Autodesk Fusion 360 part; units mm, degrees
(part 2 of 3)
  spline S12 degree 5 poles (-8.8189, 22.5399) (-8.8218, 22.5475) (-8.8279, 22.5625) (-8.8376, 22.585) (-8.8513, 22.6144) (-8.8698, 22.6507) (-8.8891, 22.6866) (-8.909, 22.7223) (-8.9293, 22.7578) (-8.9498, 22.7932) (-8.9704, 22.8286) (-8.9914, 22.8638) (-9.0127, 22.8988) (-9.0344, 22.9337) (-9.0566, 22.9684) (-9.0792, 23.0028) (-9.1021, 23.0371) (-9.1253, 23.0713) (-9.1488, 23.1053) (-9.1725, 23.1393) (-9.1964, 23.1731) (-9.2206, 23.2068) (-9.245, 23.2403) (-9.2697, 23.2738) (-9.2947, 23.3071) (-9.3199, 23.3403) (-9.3454, 23.3733) (-9.371, 23.4063) (-9.3969, 23.4391) (-9.4231, 23.4718) (-9.4494, 23.5045) (-9.4759, 23.537) (-9.5026, 23.5694) (-9.5296, 23.6016) (-9.5567, 23.6338) (-9.5841, 23.6659) (-9.6117, 23.6978) (-9.6394, 23.7297) (-9.6673, 23.7614) (-9.6955, 23.7931) (-9.7238, 23.8246) (-9.7523, 23.8561) (-9.781, 23.8874) (-9.8098, 23.9186) (-9.8389, 23.9498) (-9.8681, 23.9808) (-9.8974, 24.0117) (-9.927, 24.0425) (-9.9567, 24.0733) (-9.9866, 24.1039) (-10.0167, 24.1344) (-10.0469, 24.1649) (-10.0773, 24.1952) (-10.1079, 24.2254) (-10.1386, 24.2556) (-10.1695, 24.2856) (-10.2005, 24.3156) (-10.2317, 24.3454) (-10.263, 24.3752) (-10.2945, 24.4048) (-10.3262, 24.4344) (-10.358, 24.4639) (-10.3899, 24.4932) (-10.422, 24.5225) (-10.4543, 24.5517) (-10.4867, 24.5808) (-10.5192, 24.6098) (-10.5519, 24.6387) (-10.5847, 24.6675) (-10.6177, 24.6962) (-10.6508, 24.7248) (-10.6774, 24.7476) (-10.6974, 24.7647) (-10.7108, 24.7761) (-10.7175, 24.7818) knots 0 0 0 0 0 0 0.01428571 0.02857143 0.04285714 0.05714286 0.07142857 0.08571429 0.1 0.11428571 0.12857143 0.14285714 0.15714286 0.17142857 0.18571429 0.2 0.21428571 0.22857143 0.24285714 0.25714286 0.27142857 0.28571429 0.3 0.31428571 0.32857143 0.34285714 0.35714286 0.37142857 0.38571429 0.4 0.41428571 0.42857143 0.44285714 0.45714286 0.47142857 0.48571429 0.5 0.51428571 0.52857143 0.54285714 0.55714286 0.57142857 0.58571429 0.6 0.61428571 0.62857143 0.64285714 0.65714286 0.67142857 0.68571429 0.7 0.71428571 0.72857143 0.74285714 0.75714286 0.77142857 0.78571429 0.8 0.81428571 0.82857143 0.84285714 0.85714286 0.87142857 0.88571429 0.9 0.91428571 0.92857143 0.94285714 0.95714286 0.97142857 0.98571429 1 1 1 1 1 1
  arc A26 (-10.7175, 24.7818) -> (-12.2631, 24.0545) centre (0, 0) ccw
  spline S13 degree 5 poles (-11.7459, 21.1625) (-11.7499, 21.1696) (-11.7576, 21.184) (-11.7687, 21.2057) (-11.7827, 21.235) (-11.7989, 21.2724) (-11.8142, 21.3102) (-11.829, 21.3483) (-11.8434, 21.3865) (-11.8577, 21.4248) (-11.8717, 21.4633) (-11.8855, 21.5019) (-11.899, 21.5407) (-11.912, 21.5796) (-11.9245, 21.6188) (-11.9367, 21.6582) (-11.9485, 21.6977) (-11.96, 21.7374) (-11.9713, 21.7771) (-11.9823, 21.817) (-11.9931, 21.857) (-12.0037, 21.8971) (-12.014, 21.9374) (-12.024, 21.9777) (-12.0338, 22.0182) (-12.0433, 22.0588) (-12.0525, 22.0995) (-12.0615, 22.1402) (-12.0703, 22.1811) (-12.0789, 22.2221) (-12.0872, 22.2632) (-12.0954, 22.3043) (-12.1033, 22.3456) (-12.111, 22.3869) (-12.1185, 22.4284) (-12.1257, 22.4699) (-12.1328, 22.5115) (-12.1396, 22.5532) (-12.1463, 22.5949) (-12.1528, 22.6368) (-12.159, 22.6787) (-12.1651, 22.7207) (-12.1709, 22.7628) (-12.1766, 22.8049) (-12.1821, 22.8471) (-12.1874, 22.8894) (-12.1925, 22.9318) (-12.1974, 22.9742) (-12.2021, 23.0167) (-12.2067, 23.0592) (-12.211, 23.1019) (-12.2152, 23.1446) (-12.2192, 23.1873) (-12.223, 23.2301) (-12.2267, 23.273) (-12.2301, 23.3159) (-12.2334, 23.3589) (-12.2366, 23.402) (-12.2395, 23.4451) (-12.2423, 23.4883) (-12.2449, 23.5315) (-12.2473, 23.5748) (-12.2496, 23.6182) (-12.2517, 23.6616) (-12.2536, 23.705) (-12.2554, 23.7485) (-12.257, 23.7921) (-12.2584, 23.8357) (-12.2597, 23.8793) (-12.2608, 23.923) (-12.2617, 23.9668) (-12.2624, 24.0018) (-12.2627, 24.0281) (-12.263, 24.0457) (-12.2631, 24.0545) knots 0 0 0 0 0 0 0.01428571 0.02857143 0.04285714 0.05714286 0.07142857 0.08571429 0.1 0.11428571 0.12857143 0.14285714 0.15714286 0.17142857 0.18571429 0.2 0.21428571 0.22857143 0.24285714 0.25714286 0.27142857 0.28571429 0.3 0.31428571 0.32857143 0.34285714 0.35714286 0.37142857 0.38571429 0.4 0.41428571 0.42857143 0.44285714 0.45714286 0.47142857 0.48571429 0.5 0.51428571 0.52857143 0.54285714 0.55714286 0.57142857 0.58571429 0.6 0.61428571 0.62857143 0.64285714 0.65714286 0.67142857 0.68571429 0.7 0.71428571 0.72857143 0.74285714 0.75714286 0.77142857 0.78571429 0.8 0.81428571 0.82857143 0.84285714 0.85714286 0.87142857 0.88571429 0.9 0.91428571 0.92857143 0.94285714 0.95714286 0.97142857 0.98571429 1 1 1 1 1 1
  line L13 (-11.7459, 21.1625) -> (-11.418, 20.5712)
  arc A27 (-11.7706, 19.2333) -> (-11.418, 20.5712) centre (-12.2926, 20.0863) ccw
  arc A28 (-11.7706, 19.2333) -> (-12.3912, 18.8395) centre (0, 0) ccw
  arc A29 (-13.7518, 19.0901) -> (-12.3912, 18.8395) centre (-12.9407, 19.675) ccw
  line L14 (-13.7518, 19.0901) -> (-14.1473, 19.6386)
  spline S14 degree 5 poles (-14.1473, 19.6386) (-14.152, 19.6452) (-14.1617, 19.6583) (-14.1766, 19.6776) (-14.1972, 19.7027) (-14.2241, 19.7333) (-14.2518, 19.7632) (-14.28, 19.7928) (-14.3084, 19.8222) (-14.337, 19.8514) (-14.3658, 19.8805) (-14.3949, 19.9094) (-14.4242, 19.9381) (-14.454, 19.9664) (-14.4841, 19.9945) (-14.5145, 20.0222) (-14.5452, 20.0498) (-14.5762, 20.0771) (-14.6074, 20.1042) (-14.6388, 20.1312) (-14.6704, 20.158) (-14.7022, 20.1846) (-14.7342, 20.2111) (-14.7665, 20.2373) (-14.7989, 20.2634) (-14.8316, 20.2892) (-14.8645, 20.3149) (-14.8975, 20.3405) (-14.9308, 20.3658) (-14.9642, 20.391) (-14.9978, 20.4161) (-15.0316, 20.4409) (-15.0656, 20.4657) (-15.0997, 20.4902) (-15.134, 20.5147) (-15.1685, 20.5389) (-15.2031, 20.563) (-15.2379, 20.587) (-15.2729, 20.6108) (-15.308, 20.6344) (-15.3432, 20.6579) (-15.3787, 20.6813) (-15.4142, 20.7045) (-15.4499, 20.7276) (-15.4858, 20.7505) (-15.5218, 20.7733) (-15.558, 20.7959) (-15.5943, 20.8185) (-15.6307, 20.8408) (-15.6673, 20.8631) (-15.704, 20.8852) (-15.7408, 20.9071) (-15.7778, 20.9289) (-15.8149, 20.9506) (-15.8522, 20.9722) (-15.8896, 20.9936) (-15.9271, 21.0149) (-15.9647, 21.0361) (-16.0025, 21.0571) (-16.0403, 21.078) (-16.0783, 21.0987) (-16.1165, 21.1194) (-16.1547, 21.1399) (-16.1931, 21.1603) (-16.2316, 21.1805) (-16.2702, 21.2006) (-16.3089, 21.2206) (-16.3478, 21.2405) (-16.3867, 21.2602) (-16.4258, 21.2798) (-16.465, 21.2993) (-16.4964, 21.3148) (-16.5201, 21.3263) (-16.5359, 21.334) (-16.5438, 21.3379) knots 0 0 0 0 0 0 0.01428571 0.02857143 0.04285714 0.05714286 0.07142857 0.08571429 0.1 0.11428571 0.12857143 0.14285714 0.15714286 0.17142857 0.18571429 0.2 0.21428571 0.22857143 0.24285714 0.25714286 0.27142857 0.28571429 0.3 0.31428571 0.32857143 0.34285714 0.35714286 0.37142857 0.38571429 0.4 0.41428571 0.42857143 0.44285714 0.45714286 0.47142857 0.48571429 0.5 0.51428571 0.52857143 0.54285714 0.55714286 0.57142857 0.58571429 0.6 0.61428571 0.62857143 0.64285714 0.65714286 0.67142857 0.68571429 0.7 0.71428571 0.72857143 0.74285714 0.75714286 0.77142857 0.78571429 0.8 0.81428571 0.82857143 0.84285714 0.85714286 0.87142857 0.88571429 0.9 0.91428571 0.92857143 0.94285714 0.95714286 0.97142857 0.98571429 1 1 1 1 1 1
  arc A30 (-16.5438, 21.3379) -> (-17.8599, 20.249) centre (0, 0) ccw
  spline S15 degree 5 poles (-16.6398, 17.5766) (-16.6454, 17.5825) (-16.6564, 17.5944) (-16.6726, 17.6127) (-16.6934, 17.6377) (-16.7184, 17.6698) (-16.7427, 17.7026) (-16.7664, 17.7358) (-16.79, 17.7693) (-16.8133, 17.8029) (-16.8365, 17.8366) (-16.8594, 17.8706) (-16.8821, 17.9048) (-16.9044, 17.9393) (-16.9263, 17.9741) (-16.9479, 18.0092) (-16.9691, 18.0445) (-16.9902, 18.0801) (-17.011, 18.1158) (-17.0316, 18.1517) (-17.052, 18.1878) (-17.0722, 18.224) (-17.0922, 18.2604) (-17.1119, 18.297) (-17.1314, 18.3338) (-17.1507, 18.3707) (-17.1698, 18.4078) (-17.1886, 18.4451) (-17.2073, 18.4825) (-17.2258, 18.5201) (-17.2441, 18.5578) (-17.2622, 18.5956) (-17.2802, 18.6336) (-17.2979, 18.6717) (-17.3155, 18.71) (-17.3328, 18.7484) (-17.35, 18.7869) (-17.367, 18.8256) (-17.3838, 18.8644) (-17.4005, 18.9033) (-17.417, 18.9424) (-17.4333, 18.9815) (-17.4494, 19.0208) (-17.4654, 19.0602) (-17.4812, 19.0998) (-17.4968, 19.1394) (-17.5123, 19.1792) (-17.5276, 19.219) (-17.5428, 19.259) (-17.5578, 19.2991) (-17.5726, 19.3393) (-17.5873, 19.3796) (-17.6018, 19.42) (-17.6161, 19.4606) (-17.6303, 19.5012) (-17.6444, 19.5419) (-17.6582, 19.5828) (-17.672, 19.6237) (-17.6855, 19.6647) (-17.699, 19.7058) (-17.7122, 19.7471) (-17.7254, 19.7884) (-17.7383, 19.8298) (-17.7512, 19.8713) (-17.7638, 19.9129) (-17.7764, 19.9546) (-17.7887, 19.9964) (-17.801, 20.0383) (-17.8131, 20.0803) (-17.825, 20.1223) (-17.8368, 20.1645) (-17.8461, 20.1982) (-17.853, 20.2236) (-17.8576, 20.2406) (-17.8599, 20.249) knots 0 0 0 0 0 0 0.01428571 0.02857143 0.04285714 0.05714286 0.07142857 0.08571429 0.1 0.11428571 0.12857143 0.14285714 0.15714286 0.17142857 0.18571429 0.2 0.21428571 0.22857143 0.24285714 0.25714286 0.27142857 0.28571429 0.3 0.31428571 0.32857143 0.34285714 0.35714286 0.37142857 0.38571429 0.4 0.41428571 0.42857143 0.44285714 0.45714286 0.47142857 0.48571429 0.5 0.51428571 0.52857143 0.54285714 0.55714286 0.57142857 0.58571429 0.6 0.61428571 0.62857143 0.64285714 0.65714286 0.67142857 0.68571429 0.7 0.71428571 0.72857143 0.74285714 0.75714286 0.77142857 0.78571429 0.8 0.81428571 0.82857143 0.84285714 0.85714286 0.87142857 0.88571429 0.9 0.91428571 0.92857143 0.94285714 0.95714286 0.97142857 0.98571429 1 1 1 1 1 1
  line L15 (-16.6398, 17.5766) -> (-16.1752, 17.0854)
  arc A31 (-16.1839, 15.7018) -> (-16.1752, 17.0854) centre (-16.9016, 16.3982) ccw
  arc A32 (-16.1839, 15.7018) -> (-16.687, 15.166) centre (0, 0) ccw
  arc A33 (-18.0673, 15.0704) -> (-16.687, 15.166) centre (-17.4271, 15.8386) ccw
  line L16 (-18.0673, 15.0704) -> (-18.5867, 15.5033)
  spline S16 degree 5 poles (-18.5867, 15.5033) (-18.593, 15.5085) (-18.6056, 15.5188) (-18.6248, 15.5338) (-18.6511, 15.553) (-18.6847, 15.5759) (-18.719, 15.5981) (-18.7536, 15.6197) (-18.7884, 15.6411) (-18.8234, 15.6623) (-18.8586, 15.6833) (-18.8939, 15.7041) (-18.9295, 15.7245) (-18.9653, 15.7446) (-19.0014, 15.7643) (-19.0378, 15.7836) (-19.0744, 15.8026) (-19.1112, 15.8214) (-19.1482, 15.8399) (-19.1853, 15.8582) (-19.2226, 15.8763) (-19.26, 15.8942) (-19.2976, 15.9118) (-19.3354, 15.9293) (-19.3733, 15.9464) (-19.4114, 15.9633) (-19.4496, 15.9801) (-19.488, 15.9966) (-19.5265, 16.0128) (-19.5651, 16.0289) (-19.6039, 16.0448) (-19.6428, 16.0605) (-19.6819, 16.0761) (-19.721, 16.0914) (-19.7603, 16.1065) (-19.7997, 16.1214) (-19.8393, 16.1361) (-19.8789, 16.1507) (-19.9187, 16.165) (-19.9586, 16.1792) (-19.9986, 16.1932) (-20.0387, 16.207) (-20.079, 16.2207) (-20.1193, 16.2341) (-20.1597, 16.2474) (-20.2003, 16.2605) (-20.2409, 16.2735) (-20.2817, 16.2863) (-20.3225, 16.2989) (-20.3635, 16.3113) (-20.4046, 16.3236) (-20.4457, 16.3357) (-20.487, 16.3476) (-20.5283, 16.3594) (-20.5697, 16.371) (-20.6113, 16.3825) (-20.6529, 16.3938) (-20.6946, 16.4049) (-20.7364, 16.4159) (-20.7783, 16.4267) (-20.8203, 16.4374) (-20.8623, 16.4479) (-20.9045, 16.4582) (-20.9467, 16.4684) (-20.989, 16.4784) (-21.0314, 16.4883) (-21.0739, 16.4981) (-21.1165, 16.5076) (-21.1591, 16.5171) (-21.2018, 16.5263) (-21.2446, 16.5355) (-21.279, 16.5426) (-21.3047, 16.548) (-21.3219, 16.5515) (-21.3305, 16.5532) knots 0 0 0 0 0 0 0.01428571 0.02857143 0.04285714 0.05714286 0.07142857 0.08571429 0.1 0.11428571 0.12857143 0.14285714 0.15714286 0.17142857 0.18571429 0.2 0.21428571 0.22857143 0.24285714 0.25714286 0.27142857 0.28571429 0.3 0.31428571 0.32857143 0.34285714 0.35714286 0.37142857 0.38571429 0.4 0.41428571 0.42857143 0.44285714 0.45714286 0.47142857 0.48571429 0.5 0.51428571 0.52857143 0.54285714 0.55714286 0.57142857 0.58571429 0.6 0.61428571 0.62857143 0.64285714 0.65714286 0.67142857 0.68571429 0.7 0.71428571 0.72857143 0.74285714 0.75714286 0.77142857 0.78571429 0.8 0.81428571 0.82857143 0.84285714 0.85714286 0.87142857 0.88571429 0.9 0.91428571 0.92857143 0.94285714 0.95714286 0.97142857 0.98571429 1 1 1 1 1 1
  arc A34 (-21.3305, 16.5532) -> (-22.3345, 15.1713) centre (0, 0) ccw
  spline S17 degree 5 poles (-20.4881, 12.8862) (-20.495, 12.8906) (-20.5087, 12.8994) (-20.5289, 12.913) (-20.5553, 12.9321) (-20.5875, 12.957) (-20.6191, 12.9827) (-20.6504, 13.009) (-20.6815, 13.0355) (-20.7125, 13.0623) (-20.7433, 13.0892) (-20.774, 13.1164) (-20.8044, 13.1439) (-20.8346, 13.1717) (-20.8645, 13.2) (-20.8941, 13.2286) (-20.9235, 13.2576) (-20.9527, 13.2868) (-20.9818, 13.3162) (-21.0106, 13.3459) (-21.0394, 13.3757) (-21.068, 13.4058) (-21.0964, 13.4361) (-21.1246, 13.4666) (-21.1526, 13.4974) (-21.1805, 13.5284) (-21.2082, 13.5596) (-21.2357, 13.591) (-21.2631, 13.6226) (-21.2904, 13.6543) (-21.3175, 13.6863) (-21.3445, 13.7185) (-21.3713, 13.7508) (-21.3979, 13.7833) (-21.4244, 13.816) (-21.4508, 13.8489) (-21.477, 13.8819) (-21.5031, 13.9152) (-21.5291, 13.9486) (-21.5549, 13.9821) (-21.5806, 14.0158) (-21.6061, 14.0497) (-21.6315, 14.0838) (-21.6568, 14.118) (-21.6819, 14.1523) (-21.7069, 14.1868) (-21.7318, 14.2215) (-21.7565, 14.2563) (-21.7812, 14.2913) (-21.8057, 14.3264) (-21.83, 14.3616) (-21.8542, 14.397) (-21.8783, 14.4325) (-21.9023, 14.4682) (-21.9262, 14.504) (-21.9499, 14.54) (-21.9735, 14.5761) (-21.997, 14.6123) (-22.0203, 14.6487) (-22.0436, 14.6852) (-22.0667, 14.7218) (-22.0897, 14.7586) (-22.1125, 14.7955) (-22.1353, 14.8325) (-22.1579, 14.8696) (-22.1804, 14.9069) (-22.2028, 14.9443) (-22.225, 14.9818) (-22.2472, 15.0195) (-22.2692, 15.0572) (-22.2911, 15.0951) (-22.3085, 15.1255) (-22.3216, 15.1484) (-22.3302, 15.1637) (-22.3345, 15.1713) knots 0 0 0 0 0 0 0.01428571 0.02857143 0.04285714 0.05714286 0.07142857 0.08571429 0.1 0.11428571 0.12857143 0.14285714 0.15714286 0.17142857 0.18571429 0.2 0.21428571 0.22857143 0.24285714 0.25714286 0.27142857 0.28571429 0.3 0.31428571 0.32857143 0.34285714 0.35714286 0.37142857 0.38571429 0.4 0.41428571 0.42857143 0.44285714 0.45714286 0.47142857 0.48571429 0.5 0.51428571 0.52857143 0.54285714 0.55714286 0.57142857 0.58571429 0.6 0.61428571 0.62857143 0.64285714 0.65714286 0.67142857 0.68571429 0.7 0.71428571 0.72857143 0.74285714 0.75714286 0.77142857 0.78571429 0.8 0.81428571 0.82857143 0.84285714 0.85714286 0.87142857 0.88571429 0.9 0.91428571 0.92857143 0.94285714 0.95714286 0.97142857 0.98571429 1 1 1 1 1 1
  line L17 (-20.4881, 12.8862) -> (-19.9159, 12.526)
  arc A35 (-19.5803, 11.1838) -> (-19.9159, 12.526) centre (-20.4487, 11.6797) ccw
  arc A36 (-19.5803, 11.1838) -> (-19.9344, 10.5397) centre (0, 0) ccw
  arc A37 (-21.2476, 10.1038) -> (-19.9344, 10.5397) centre (-20.8185, 11.0071) ccw
  line L18 (-21.2476, 10.1038) -> (-21.8583, 10.3939)
  spline S18 degree 5 poles (-21.8583, 10.3939) (-21.8656, 10.3974) (-21.8804, 10.4042) (-21.9028, 10.414) (-21.933, 10.4261) (-21.9713, 10.4399) (-22.0099, 10.4528) (-22.0489, 10.4652) (-22.088, 10.4772) (-22.1271, 10.489) (-22.1664, 10.5006) (-22.2058, 10.512) (-22.2453, 10.5229) (-22.285, 10.5335) (-22.3249, 10.5435) (-22.3649, 10.5532) (-22.4051, 10.5625) (-22.4454, 10.5715) (-22.4859, 10.5803) (-22.5264, 10.5888) (-22.567, 10.5971) (-22.6077, 10.6051) (-22.6484, 10.6128) (-22.6893, 10.6203) (-22.7303, 10.6275) (-22.7714, 10.6344) (-22.8126, 10.6411) (-22.8539, 10.6475) (-22.8953, 10.6537) (-22.9367, 10.6597) (-22.9782, 10.6655) (-23.0198, 10.671) (-23.0615, 10.6763) (-23.1032, 10.6814) (-23.145, 10.6863) (-23.1869, 10.6909) (-23.2289, 10.6953) (-23.2709, 10.6996) (-23.313, 10.7036) (-23.3552, 10.7074) (-23.3974, 10.711) (-23.4397, 10.7144) (-23.4821, 10.7176) (-23.5245, 10.7206) (-23.5669, 10.7235) (-23.6095, 10.7261) (-23.6521, 10.7285) (-23.6947, 10.7308) (-23.7374, 10.7328) (-23.7802, 10.7347) (-23.823, 10.7363) (-23.8659, 10.7378) (-23.9088, 10.7392) (-23.9518, 10.7403) (-23.9948, 10.7412) (-24.0379, 10.742) (-24.081, 10.7426) (-24.1242, 10.743) (-24.1674, 10.7432) (-24.2107, 10.7433) (-24.254, 10.7432) (-24.2973, 10.7429) (-24.3407, 10.7424) (-24.3842, 10.7418) (-24.4276, 10.741) (-24.4712, 10.74) (-24.5147, 10.7389) (-24.5583, 10.7376) (-24.602, 10.7361) (-24.6457, 10.7344) (-24.6894, 10.7326) (-24.7244, 10.7311) (-24.7507, 10.7298) (-24.7682, 10.7289) (-24.777, 10.7285) knots 0 0 0 0 0 0 0.01428571 0.02857143 0.04285714 0.05714286 0.07142857 0.08571429 0.1 0.11428571 0.12857143 0.14285714 0.15714286 0.17142857 0.18571429 0.2 0.21428571 0.22857143 0.24285714 0.25714286 0.27142857 0.28571429 0.3 0.31428571 0.32857143 0.34285714 0.35714286 0.37142857 0.38571429 0.4 0.41428571 0.42857143 0.44285714 0.45714286 0.47142857 0.48571429 0.5 0.51428571 0.52857143 0.54285714 0.55714286 0.57142857 0.58571429 0.6 0.61428571 0.62857143 0.64285714 0.65714286 0.67142857 0.68571429 0.7 0.71428571 0.72857143 0.74285714 0.75714286 0.77142857 0.78571429 0.8 0.81428571 0.82857143 0.84285714 0.85714286 0.87142857 0.88571429 0.9 0.91428571 0.92857143 0.94285714 0.95714286 0.97142857 0.98571429 1 1 1 1 1 1
  arc A38 (-24.777, 10.7285) -> (-25.4058, 9.1403) centre (0, 0) ccw
  spline S19 degree 5 poles (-23.0491, 7.3862) (-23.0569, 7.3887) (-23.0723, 7.3938) (-23.0953, 7.402) (-23.1256, 7.4139) (-23.163, 7.43) (-23.2, 7.4471) (-23.2368, 7.4647) (-23.2736, 7.4827) (-23.3102, 7.5009) (-23.3468, 7.5193) (-23.3832, 7.538) (-23.4196, 7.5571) (-23.4557, 7.5766) (-23.4917, 7.5965) (-23.5275, 7.6169) (-23.5632, 7.6376) (-23.5987, 7.6586) (-23.6342, 7.6799) (-23.6695, 7.7015) (-23.7048, 7.7232) (-23.7399, 7.7452) (-23.775, 7.7675) (-23.8099, 7.7901) (-23.8447, 7.8129) (-23.8794, 7.836) (-23.914, 7.8593) (-23.9485, 7.8829) (-23.9829, 7.9066) (-24.0172, 7.9307) (-24.0514, 7.9549) (-24.0855, 7.9793) (-24.1195, 8.004) (-24.1534, 8.0288) (-24.1873, 8.0539) (-24.221, 8.0792) (-24.2546, 8.1047) (-24.2881, 8.1304) (-24.3216, 8.1563) (-24.3549, 8.1824) (-24.3882, 8.2086) (-24.4213, 8.2351) (-24.4544, 8.2618) (-24.4874, 8.2886) (-24.5203, 8.3156) (-24.5531, 8.3428) (-24.5858, 8.3702) (-24.6184, 8.3978) (-24.651, 8.4255) (-24.6834, 8.4534) (-24.7158, 8.4815) (-24.748, 8.5098) (-24.7802, 8.5382) (-24.8123, 8.5668) (-24.8443, 8.5956) (-24.8763, 8.6245) (-24.9081, 8.6536) (-24.9398, 8.6828) (-24.9715, 8.7122) (-25.0031, 8.7418) (-25.0346, 8.7715) (-25.066, 8.8014) (-25.0973, 8.8315) (-25.1285, 8.8617) (-25.1597, 8.892) (-25.1908, 8.9225) (-25.2217, 8.9532) (-25.2526, 8.984) (-25.2834, 9.015) (-25.3142, 9.0461) (-25.3448, 9.0773) (-25.3693, 9.1024) (-25.3875, 9.1213) (-25.3997, 9.134) (-25.4058, 9.1403) knots 0 0 0 0 0 0 0.01428571 0.02857143 0.04285714 0.05714286 0.07142857 0.08571429 0.1 0.11428571 0.12857143 0.14285714 0.15714286 0.17142857 0.18571429 0.2 0.21428571 0.22857143 0.24285714 0.25714286 0.27142857 0.28571429 0.3 0.31428571 0.32857143 0.34285714 0.35714286 0.37142857 0.38571429 0.4 0.41428571 0.42857143 0.44285714 0.45714286 0.47142857 0.48571429 0.5 0.51428571 0.52857143 0.54285714 0.55714286 0.57142857 0.58571429 0.6 0.61428571 0.62857143 0.64285714 0.65714286 0.67142857 0.68571429 0.7 0.71428571 0.72857143 0.74285714 0.75714286 0.77142857 0.78571429 0.8 0.81428571 0.82857143 0.84285714 0.85714286 0.87142857 0.88571429 0.9 0.91428571 0.92857143 0.94285714 0.95714286 0.97142857 0.98571429 1 1 1 1 1 1
  line L19 (-23.0491, 7.3862) -> (-22.4053, 7.1796)
  arc A39 (-21.7465, 5.963) -> (-22.4053, 7.1796) centre (-22.7109, 6.2274) ccw
  arc A40 (-21.7465, 5.963) -> (-21.9293, 5.2511) centre (0, 0) ccw
  arc A41 (-23.0927, 4.5023) -> (-21.9293, 5.2511) centre (-22.9018, 5.4839) ccw
  line L20 (-23.0927, 4.5023) -> (-23.7564, 4.6314)
  spline S20 degree 5 poles (-23.7564, 4.6314) (-23.7644, 4.633) (-23.7804, 4.6359) (-23.8045, 4.6398) (-23.8368, 4.644) (-23.8773, 4.6479) (-23.918, 4.6508) (-23.9588, 4.653) (-23.9996, 4.655) (-24.0405, 4.6567) (-24.0814, 4.6582) (-24.1223, 4.6594) (-24.1634, 4.6602) (-24.2044, 4.6605) (-24.2456, 4.6603) (-24.2868, 4.6597) (-24.328, 4.6588) (-24.3693, 4.6575) (-24.4106, 4.6559) (-24.452, 4.6541) (-24.4934, 4.652) (-24.5348, 4.6496) (-24.5762, 4.647) (-24.6177, 4.644) (-24.6592, 4.6408) (-24.7007, 4.6373) (-24.7423, 4.6335) (-24.7838, 4.6295) (-24.8254, 4.6252) (-24.8671, 4.6207) (-24.9087, 4.6159) (-24.9504, 4.611) (-24.992, 4.6057) (-25.0337, 4.6003) (-25.0755, 4.5946) (-25.1172, 4.5887) (-25.1589, 4.5825) (-25.2007, 4.5762) (-25.2425, 4.5696) (-25.2843, 4.5628) (-25.3261, 4.5558) (-25.3679, 4.5486) (-25.4097, 4.5412) (-25.4515, 4.5335) (-25.4934, 4.5257) (-25.5352, 4.5177) (-25.5771, 4.5094) (-25.6189, 4.501) (-25.6608, 4.4924) (-25.7027, 4.4835) (-25.7446, 4.4745) (-25.7865, 4.4653) (-25.8284, 4.4559) (-25.8703, 4.4463) (-25.9122, 4.4365) (-25.9541, 4.4265) (-25.996, 4.4164) (-26.0379, 4.406) (-26.0799, 4.3955) (-26.1218, 4.3848) (-26.1637, 4.3739) (-26.2056, 4.3629) (-26.2475, 4.3516) (-26.2895, 4.3402) (-26.3314, 4.3286) (-26.3733, 4.3169) (-26.4152, 4.3049) (-26.4571, 4.2928) (-26.499, 4.2805) (-26.5409, 4.2681) (-26.5828, 4.2555) (-26.6164, 4.2452) (-26.6415, 4.2375) (-26.6583, 4.2323) (-26.6666, 4.2297) knots 0 0 0 0 0 0 0.01428571 0.02857143 0.04285714 0.05714286 0.07142857 0.08571429 0.1 0.11428571 0.12857143 0.14285714 0.15714286 0.17142857 0.18571429 0.2 0.21428571 0.22857143 0.24285714 0.25714286 0.27142857 0.28571429 0.3 0.31428571 0.32857143 0.34285714 0.35714286 0.37142857 0.38571429 0.4 0.41428571 0.42857143 0.44285714 0.45714286 0.47142857 0.48571429 0.5 0.51428571 0.52857143 0.54285714 0.55714286 0.57142857 0.58571429 0.6 0.61428571 0.62857143 0.64285714 0.65714286 0.67142857 0.68571429 0.7 0.71428571 0.72857143 0.74285714 0.75714286 0.77142857 0.78571429 0.8 0.81428571 0.82857143 0.84285714 0.85714286 0.87142857 0.88571429 0.9 0.91428571 0.92857143 0.94285714 0.95714286 0.97142857 0.98571429 1 1 1 1 1 1
  arc A42 (-26.6666, 4.2297) -> (-26.8807, 2.535) centre (0, 0) ccw
  spline S21 degree 5 poles (-24.1619, 1.422) (-24.17, 1.4225) (-24.1862, 1.4237) (-24.2105, 1.4259) (-24.2428, 1.4299) (-24.283, 1.4362) (-24.3231, 1.4435) (-24.3632, 1.4514) (-24.4032, 1.4597) (-24.4433, 1.4682) (-24.4833, 1.477) (-24.5232, 1.486) (-24.5632, 1.4954) (-24.603, 1.5053) (-24.6428, 1.5157) (-24.6826, 1.5265) (-24.7223, 1.5377) (-24.762, 1.5493) (-24.8016, 1.5611) (-24.8412, 1.5731) (-24.8808, 1.5854) (-24.9203, 1.598) (-24.9598, 1.6109) (-24.9992, 1.624) (-25.0386, 1.6375) (-25.0779, 1.6512) (-25.1172, 1.6652) (-25.1565, 1.6795) (-25.1957, 1.6939) (-25.2349, 1.7087) (-25.2741, 1.7236) (-25.3132, 1.7388) (-25.3523, 1.7542) (-25.3913, 1.7699) (-25.4303, 1.7858) (-25.4692, 1.8019) (-25.5082, 1.8182) (-25.547, 1.8347) (-25.5858, 1.8515) (-25.6246, 1.8685) (-25.6634, 1.8857) (-25.7021, 1.903) (-25.7407, 1.9206) (-25.7794, 1.9384) (-25.8179, 1.9564) (-25.8565, 1.9746) (-25.895, 1.993) (-25.9334, 2.0116) (-25.9718, 2.0304) (-26.0102, 2.0493) (-26.0485, 2.0685) (-26.0868, 2.0878) (-26.1251, 2.1074) (-26.1633, 2.1271) (-26.2014, 2.147) (-26.2395, 2.1671) (-26.2776, 2.1873) (-26.3156, 2.2078) (-26.3536, 2.2284) (-26.3916, 2.2492) (-26.4295, 2.2701) (-26.4673, 2.2913) (-26.5051, 2.3126) (-26.5429, 2.3341) (-26.5806, 2.3557) (-26.6183, 2.3775) (-26.6559, 2.3995) (-26.6935, 2.4217) (-26.731, 2.444) (-26.7685, 2.4665) (-26.806, 2.4891) (-26.8359, 2.5074) (-26.8583, 2.5211) (-26.8733, 2.5303) (-26.8807, 2.535) knots 0 0 0 0 0 0 0.01428571 0.02857143 0.04285714 0.05714286 0.07142857 0.08571429 0.1 0.11428571 0.12857143 0.14285714 0.15714286 0.17142857 0.18571429 0.2 0.21428571 0.22857143 0.24285714 0.25714286 0.27142857 0.28571429 0.3 0.31428571 0.32857143 0.34285714 0.35714286 0.37142857 0.38571429 0.4 0.41428571 0.42857143 0.44285714 0.45714286 0.47142857 0.48571429 0.5 0.51428571 0.52857143 0.54285714 0.55714286 0.57142857 0.58571429 0.6 0.61428571 0.62857143 0.64285714 0.65714286 0.67142857 0.68571429 0.7 0.71428571 0.72857143 0.74285714 0.75714286 0.77142857 0.78571429 0.8 0.81428571 0.82857143 0.84285714 0.85714286 0.87142857 0.88571429 0.9 0.91428571 0.92857143 0.94285714 0.95714286 0.97142857 0.98571429 1 1 1 1 1 1
  line L21 (-24.1619, 1.422) -> (-23.4869, 1.382)
  arc A43 (-22.5462, 0.3675) -> (-23.4869, 1.382) centre (-23.5461, 0.3838) ccw
  arc A44 (-22.5462, 0.3675) -> (-22.5462, -0.3675) centre (0, 0) ccw
  arc A45 (-23.4869, -1.382) -> (-22.5462, -0.3675) centre (-23.5461, -0.3838) ccw
  line L22 (-23.4869, -1.382) -> (-24.1619, -1.422)
  spline S22 degree 5 poles (-24.1619, -1.422) (-24.17, -1.4225) (-24.1862, -1.4237) (-24.2105, -1.4259) (-24.2428, -1.4299) (-24.283, -1.4362) (-24.3231, -1.4435) (-24.3632, -1.4514) (-24.4032, -1.4597) (-24.4433, -1.4682) (-24.4833, -1.477) (-24.5232, -1.486) (-24.5632, -1.4954) (-24.603, -1.5053) (-24.6428, -1.5157) (-24.6826, -1.5265) (-24.7223, -1.5377) (-24.762, -1.5493) (-24.8016, -1.5611) (-24.8412, -1.5731) (-24.8808, -1.5854) (-24.9203, -1.598) (-24.9598, -1.6109) (-24.9992, -1.624) (-25.0386, -1.6375) (-25.0779, -1.6512) (-25.1172, -1.6652) (-25.1565, -1.6795) (-25.1957, -1.6939) (-25.2349, -1.7087) (-25.2741, -1.7236) (-25.3132, -1.7388) (-25.3523, -1.7542) (-25.3913, -1.7699) (-25.4303, -1.7858) (-25.4692, -1.8019) (-25.5082, -1.8182) (-25.547, -1.8347) (-25.5858, -1.8515) (-25.6246, -1.8685) (-25.6634, -1.8857) (-25.7021, -1.903) (-25.7407, -1.9206) (-25.7794, -1.9384) (-25.8179, -1.9564) (-25.8565, -1.9746) (-25.895, -1.993) (-25.9334, -2.0116) (-25.9718, -2.0304) (-26.0102, -2.0493) (-26.0485, -2.0685) (-26.0868, -2.0878) (-26.1251, -2.1074) (-26.1633, -2.1271) (-26.2014, -2.147) (-26.2395, -2.1671) (-26.2776, -2.1873) (-26.3156, -2.2078) (-26.3536, -2.2284) (-26.3916, -2.2492) (-26.4295, -2.2701) (-26.4673, -2.2913) (-26.5051, -2.3126) (-26.5429, -2.3341) (-26.5806, -2.3557) (-26.6183, -2.3775) (-26.6559, -2.3995) (-26.6935, -2.4217) (-26.731, -2.444) (-26.7685, -2.4665) (-26.806, -2.4891) (-26.8359, -2.5074) (-26.8583, -2.5211) (-26.8733, -2.5303) (-26.8807, -2.535) knots 0 0 0 0 0 0 0.01428571 0.02857143 0.04285714 0.05714286 0.07142857 0.08571429 0.1 0.11428571 0.12857143 0.14285714 0.15714286 0.17142857 0.18571429 0.2 0.21428571 0.22857143 0.24285714 0.25714286 0.27142857 0.28571429 0.3 0.31428571 0.32857143 0.34285714 0.35714286 0.37142857 0.38571429 0.4 0.41428571 0.42857143 0.44285714 0.45714286 0.47142857 0.48571429 0.5 0.51428571 0.52857143 0.54285714 0.55714286 0.57142857 0.58571429 0.6 0.61428571 0.62857143 0.64285714 0.65714286 0.67142857 0.68571429 0.7 0.71428571 0.72857143 0.74285714 0.75714286 0.77142857 0.78571429 0.8 0.81428571 0.82857143 0.84285714 0.85714286 0.87142857 0.88571429 0.9 0.91428571 0.92857143 0.94285714 0.95714286 0.97142857 0.98571429 1 1 1 1 1 1
  arc A46 (-26.8807, -2.535) -> (-26.6666, -4.2297) centre (0, 0) ccw
  spline S23 degree 5 poles (-23.7564, -4.6314) (-23.7644, -4.633) (-23.7804, -4.6359) (-23.8045, -4.6398) (-23.8368, -4.644) (-23.8773, -4.6479) (-23.918, -4.6508) (-23.9588, -4.653) (-23.9996, -4.655) (-24.0405, -4.6567) (-24.0814, -4.6582) (-24.1223, -4.6594) (-24.1634, -4.6602) (-24.2044, -4.6605) (-24.2456, -4.6603) (-24.2868, -4.6597) (-24.328, -4.6588) (-24.3693, -4.6575) (-24.4106, -4.6559) (-24.452, -4.6541) (-24.4934, -4.652) (-24.5348, -4.6496) (-24.5762, -4.647) (-24.6177, -4.644) (-24.6592, -4.6408) (-24.7007, -4.6373) (-24.7423, -4.6335) (-24.7838, -4.6295) (-24.8254, -4.6252) (-24.8671, -4.6207) (-24.9087, -4.6159) (-24.9504, -4.611) (-24.992, -4.6057) (-25.0337, -4.6003) (-25.0755, -4.5946) (-25.1172, -4.5887) (-25.1589, -4.5825) (-25.2007, -4.5762) (-25.2425, -4.5696) (-25.2843, -4.5628) (-25.3261, -4.5558) (-25.3679, -4.5486) (-25.4097, -4.5412) (-25.4515, -4.5335) (-25.4934, -4.5257) (-25.5352, -4.5177) (-25.5771, -4.5094) (-25.6189, -4.501) (-25.6608, -4.4924) (-25.7027, -4.4835) (-25.7446, -4.4745) (-25.7865, -4.4653) (-25.8284, -4.4559) (-25.8703, -4.4463) (-25.9122, -4.4365) (-25.9541, -4.4265) (-25.996, -4.4164) (-26.0379, -4.406) (-26.0799, -4.3955) (-26.1218, -4.3848) (-26.1637, -4.3739) (-26.2056, -4.3629) (-26.2475, -4.3516) (-26.2895, -4.3402) (-26.3314, -4.3286) (-26.3733, -4.3169) (-26.4152, -4.3049) (-26.4571, -4.2928) (-26.499, -4.2805) (-26.5409, -4.2681) (-26.5828, -4.2555) (-26.6164, -4.2452) (-26.6415, -4.2375) (-26.6583, -4.2323) (-26.6666, -4.2297) knots 0 0 0 0 0 0 0.01428571 0.02857143 0.04285714 0.05714286 0.07142857 0.08571429 0.1 0.11428571 0.12857143 0.14285714 0.15714286 0.17142857 0.18571429 0.2 0.21428571 0.22857143 0.24285714 0.25714286 0.27142857 0.28571429 0.3 0.31428571 0.32857143 0.34285714 0.35714286 0.37142857 0.38571429 0.4 0.41428571 0.42857143 0.44285714 0.45714286 0.47142857 0.48571429 0.5 0.51428571 0.52857143 0.54285714 0.55714286 0.57142857 0.58571429 0.6 0.61428571 0.62857143 0.64285714 0.65714286 0.67142857 0.68571429 0.7 0.71428571 0.72857143 0.74285714 0.75714286 0.77142857 0.78571429 0.8 0.81428571 0.82857143 0.84285714 0.85714286 0.87142857 0.88571429 0.9 0.91428571 0.92857143 0.94285714 0.95714286 0.97142857 0.98571429 1 1 1 1 1 1
  line L23 (-23.7564, -4.6314) -> (-23.0927, -4.5023)
  arc A47 (-21.9293, -5.2511) -> (-23.0927, -4.5023) centre (-22.9018, -5.4839) ccw
  arc A48 (-21.9293, -5.2511) -> (-21.7465, -5.963) centre (0, 0) ccw
  arc A49 (-22.4053, -7.1796) -> (-21.7465, -5.963) centre (-22.7109, -6.2274) ccw
  line L24 (-22.4053, -7.1796) -> (-23.0491, -7.3862)
  spline S24 degree 5 poles (-23.0491, -7.3862) (-23.0569, -7.3887) (-23.0723, -7.3938) (-23.0953, -7.402) (-23.1256, -7.4139) (-23.163, -7.43) (-23.2, -7.4471) (-23.2368, -7.4647) (-23.2736, -7.4827) (-23.3102, -7.5009) (-23.3468, -7.5193) (-23.3832, -7.538) (-23.4196, -7.5571) (-23.4557, -7.5766) (-23.4917, -7.5965) (-23.5275, -7.6169) (-23.5632, -7.6376) (-23.5987, -7.6586) (-23.6342, -7.6799) (-23.6695, -7.7015) (-23.7048, -7.7232) (-23.7399, -7.7452) (-23.775, -7.7675) (-23.8099, -7.7901) (-23.8447, -7.8129) (-23.8794, -7.836) (-23.914, -7.8593) (-23.9485, -7.8829) (-23.9829, -7.9066) (-24.0172, -7.9307) (-24.0514, -7.9549) (-24.0855, -7.9793) (-24.1195, -8.004) (-24.1534, -8.0288) (-24.1873, -8.0539) (-24.221, -8.0792) (-24.2546, -8.1047) (-24.2881, -8.1304) (-24.3216, -8.1563) (-24.3549, -8.1824) (-24.3882, -8.2086) (-24.4213, -8.2351) (-24.4544, -8.2618) (-24.4874, -8.2886) (-24.5203, -8.3156) (-24.5531, -8.3428) (-24.5858, -8.3702) (-24.6184, -8.3978) (-24.651, -8.4255) (-24.6834, -8.4534) (-24.7158, -8.4815) (-24.748, -8.5098) (-24.7802, -8.5382) (-24.8123, -8.5668) (-24.8443, -8.5956) (-24.8763, -8.6245) (-24.9081, -8.6536) (-24.9398, -8.6828) (-24.9715, -8.7122) (-25.0031, -8.7418) (-25.0346, -8.7715) (-25.066, -8.8014) (-25.0973, -8.8315) (-25.1285, -8.8617) (-25.1597, -8.892) (-25.1908, -8.9225) (-25.2217, -8.9532) (-25.2526, -8.984) (-25.2834, -9.015) (-25.3142, -9.0461) (-25.3448, -9.0773) (-25.3693, -9.1024) (-25.3875, -9.1213) (-25.3997, -9.134) (-25.4058, -9.1403) knots 0 0 0 0 0 0 0.01428571 0.02857143 0.04285714 0.05714286 0.07142857 0.08571429 0.1 0.11428571 0.12857143 0.14285714 0.15714286 0.17142857 0.18571429 0.2 0.21428571 0.22857143 0.24285714 0.25714286 0.27142857 0.28571429 0.3 0.31428571 0.32857143 0.34285714 0.35714286 0.37142857 0.38571429 0.4 0.41428571 0.42857143 0.44285714 0.45714286 0.47142857 0.48571429 0.5 0.51428571 0.52857143 0.54285714 0.55714286 0.57142857 0.58571429 0.6 0.61428571 0.62857143 0.64285714 0.65714286 0.67142857 0.68571429 0.7 0.71428571 0.72857143 0.74285714 0.75714286 0.77142857 0.78571429 0.8 0.81428571 0.82857143 0.84285714 0.85714286 0.87142857 0.88571429 0.9 0.91428571 0.92857143 0.94285714 0.95714286 0.97142857 0.98571429 1 1 1 1 1 1
  arc A50 (-25.4058, -9.1403) -> (-24.777, -10.7285) centre (0, 0) ccw
  spline S25 degree 5 poles (-21.8583, -10.3939) (-21.8656, -10.3974) (-21.8804, -10.4042) (-21.9028, -10.414) (-21.933, -10.4261) (-21.9713, -10.4399) (-22.0099, -10.4528) (-22.0489, -10.4652) (-22.088, -10.4772) (-22.1271, -10.489) (-22.1664, -10.5006) (-22.2058, -10.512) (-22.2453, -10.5229) (-22.285, -10.5335) (-22.3249, -10.5435) (-22.3649, -10.5532) (-22.4051, -10.5625) (-22.4454, -10.5715) (-22.4859, -10.5803) (-22.5264, -10.5888) (-22.567, -10.5971) (-22.6077, -10.6051) (-22.6484, -10.6128) (-22.6893, -10.6203) (-22.7303, -10.6275) (-22.7714, -10.6344) (-22.8126, -10.6411) (-22.8539, -10.6475) (-22.8953, -10.6537) (-22.9367, -10.6597) (-22.9782, -10.6655) (-23.0198, -10.671) (-23.0615, -10.6763) (-23.1032, -10.6814) (-23.145, -10.6863) (-23.1869, -10.6909) (-23.2289, -10.6953) (-23.2709, -10.6996) (-23.313, -10.7036) (-23.3552, -10.7074) (-23.3974, -10.711) (-23.4397, -10.7144) (-23.4821, -10.7176) (-23.5245, -10.7206) (-23.5669, -10.7235) (-23.6095, -10.7261) (-23.6521, -10.7285) (-23.6947, -10.7308) (-23.7374, -10.7328) (-23.7802, -10.7347) (-23.823, -10.7363) (-23.8659, -10.7378) (-23.9088, -10.7391) (-23.9518, -10.7403) (-23.9948, -10.7412) (-24.0379, -10.742) (-24.081, -10.7426) (-24.1242, -10.743) (-24.1674, -10.7432) (-24.2107, -10.7433) (-24.254, -10.7432) (-24.2973, -10.7429) (-24.3407, -10.7424) (-24.3842, -10.7418) (-24.4276, -10.741) (-24.4712, -10.74) (-24.5147, -10.7389) (-24.5583, -10.7376) (-24.602, -10.7361) (-24.6457, -10.7344) (-24.6894, -10.7326) (-24.7244, -10.7311) (-24.7507, -10.7298) (-24.7682, -10.7289) (-24.777, -10.7285) knots 0 0 0 0 0 0 0.01428571 0.02857143 0.04285714 0.05714286 0.07142857 0.08571429 0.1 0.11428571 0.12857143 0.14285714 0.15714286 0.17142857 0.18571429 0.2 0.21428571 0.22857143 0.24285714 0.25714286 0.27142857 0.28571429 0.3 0.31428571 0.32857143 0.34285714 0.35714286 0.37142857 0.38571429 0.4 0.41428571 0.42857143 0.44285714 0.45714286 0.47142857 0.48571429 0.5 0.51428571 0.52857143 0.54285714 0.55714286 0.57142857 0.58571429 0.6 0.61428571 0.62857143 0.64285714 0.65714286 0.67142857 0.68571429 0.7 0.71428571 0.72857143 0.74285714 0.75714286 0.77142857 0.78571429 0.8 0.81428571 0.82857143 0.84285714 0.85714286 0.87142857 0.88571429 0.9 0.91428571 0.92857143 0.94285714 0.95714286 0.97142857 0.98571429 1 1 1 1 1 1
  line L25 (-21.8583, -10.3939) -> (-21.2476, -10.1038)
  arc A51 (-19.9344, -10.5397) -> (-21.2476, -10.1038) centre (-20.8185, -11.0071) ccw
  arc A52 (-19.9344, -10.5397) -> (-19.5803, -11.1838) centre (0, 0) ccw
  arc A53 (-19.9159, -12.526) -> (-19.5803, -11.1838) centre (-20.4487, -11.6797) ccw
  line L26 (-19.9159, -12.526) -> (-20.4881, -12.8862)
  spline S26 degree 5 poles (-20.4881, -12.8862) (-20.495, -12.8906) (-20.5087, -12.8994) (-20.5289, -12.913) (-20.5553, -12.9321) (-20.5875, -12.957) (-20.6191, -12.9827) (-20.6504, -13.009) (-20.6815, -13.0355) (-20.7125, -13.0623) (-20.7433, -13.0892) (-20.774, -13.1164) (-20.8044, -13.1439) (-20.8346, -13.1717) (-20.8645, -13.2) (-20.8941, -13.2286) (-20.9235, -13.2576) (-20.9527, -13.2868) (-20.9818, -13.3162) (-21.0106, -13.3459) (-21.0394, -13.3757) (-21.068, -13.4058) (-21.0964, -13.4361) (-21.1246, -13.4666) (-21.1526, -13.4974) (-21.1805, -13.5284) (-21.2082, -13.5596) (-21.2357, -13.591) (-21.2631, -13.6226) (-21.2904, -13.6543) (-21.3175, -13.6863) (-21.3445, -13.7185) (-21.3713, -13.7508) (-21.3979, -13.7833) (-21.4244, -13.816) (-21.4508, -13.8489) (-21.477, -13.8819) (-21.5031, -13.9152) (-21.5291, -13.9486) (-21.5549, -13.9821) (-21.5806, -14.0158) (-21.6061, -14.0497) (-21.6315, -14.0838) (-21.6568, -14.118) (-21.6819, -14.1523) (-21.7069, -14.1868) (-21.7318, -14.2215) (-21.7565, -14.2563) (-21.7812, -14.2913) (-21.8057, -14.3264) (-21.83, -14.3616) (-21.8542, -14.397) (-21.8783, -14.4325) (-21.9023, -14.4682) (-21.9262, -14.504) (-21.9499, -14.54) (-21.9735, -14.5761) (-21.997, -14.6123) (-22.0203, -14.6487) (-22.0436, -14.6852) (-22.0667, -14.7218) (-22.0897, -14.7586) (-22.1125, -14.7955) (-22.1353, -14.8325) (-22.1579, -14.8696) (-22.1804, -14.9069) (-22.2028, -14.9443) (-22.225, -14.9818) (-22.2472, -15.0195) (-22.2692, -15.0572) (-22.2911, -15.0951) (-22.3085, -15.1255) (-22.3216, -15.1484) (-22.3302, -15.1637) (-22.3345, -15.1713) knots 0 0 0 0 0 0 0.01428571 0.02857143 0.04285714 0.05714286 0.07142857 0.08571429 0.1 0.11428571 0.12857143 0.14285714 0.15714286 0.17142857 0.18571429 0.2 0.21428571 0.22857143 0.24285714 0.25714286 0.27142857 0.28571429 0.3 0.31428571 0.32857143 0.34285714 0.35714286 0.37142857 0.38571429 0.4 0.41428571 0.42857143 0.44285714 0.45714286 0.47142857 0.48571429 0.5 0.51428571 0.52857143 0.54285714 0.55714286 0.57142857 0.58571429 0.6 0.61428571 0.62857143 0.64285714 0.65714286 0.67142857 0.68571429 0.7 0.71428571 0.72857143 0.74285714 0.75714286 0.77142857 0.78571429 0.8 0.81428571 0.82857143 0.84285714 0.85714286 0.87142857 0.88571429 0.9 0.91428571 0.92857143 0.94285714 0.95714286 0.97142857 0.98571429 1 1 1 1 1 1
  arc A54 (-22.3345, -15.1713) -> (-21.3305, -16.5532) centre (0, 0) ccw
  spline S27 degree 5 poles (-18.5867, -15.5033) (-18.593, -15.5085) (-18.6056, -15.5188) (-18.6248, -15.5338) (-18.6511, -15.553) (-18.6847, -15.5759) (-18.719, -15.5981) (-18.7536, -15.6197) (-18.7884, -15.6411) (-18.8234, -15.6623) (-18.8586, -15.6833) (-18.8939, -15.7041) (-18.9295, -15.7245) (-18.9653, -15.7446) (-19.0014, -15.7643) (-19.0378, -15.7836) (-19.0744, -15.8026) (-19.1112, -15.8214) (-19.1482, -15.8399) (-19.1853, -15.8582) (-19.2226, -15.8763) (-19.26, -15.8942) (-19.2976, -15.9118) (-19.3354, -15.9293) (-19.3733, -15.9464) (-19.4114, -15.9633) (-19.4496, -15.9801) (-19.488, -15.9966) (-19.5265, -16.0128) (-19.5651, -16.0289) (-19.6039, -16.0448) (-19.6428, -16.0605) (-19.6819, -16.0761) (-19.721, -16.0914) (-19.7603, -16.1065) (-19.7997, -16.1214) (-19.8393, -16.1361) (-19.8789, -16.1507) (-19.9187, -16.165) (-19.9586, -16.1792) (-19.9986, -16.1932) (-20.0387, -16.207) (-20.079, -16.2207) (-20.1193, -16.2341) (-20.1597, -16.2474) (-20.2003, -16.2605) (-20.2409, -16.2735) (-20.2817, -16.2863) (-20.3225, -16.2989) (-20.3635, -16.3113) (-20.4046, -16.3236) (-20.4457, -16.3357) (-20.487, -16.3476) (-20.5283, -16.3594) (-20.5697, -16.371) (-20.6113, -16.3825) (-20.6529, -16.3938) (-20.6946, -16.4049) (-20.7364, -16.4159) (-20.7783, -16.4267) (-20.8203, -16.4374) (-20.8623, -16.4479) (-20.9045, -16.4582) (-20.9467, -16.4684) (-20.989, -16.4784) (-21.0314, -16.4883) (-21.0739, -16.4981) (-21.1165, -16.5076) (-21.1591, -16.5171) (-21.2018, -16.5263) (-21.2446, -16.5355) (-21.279, -16.5426) (-21.3047, -16.548) (-21.3219, -16.5515) (-21.3305, -16.5532) knots 0 0 0 0 0 0 0.01428571 0.02857143 0.04285714 0.05714286 0.07142857 0.08571429 0.1 0.11428571 0.12857143 0.14285714 0.15714286 0.17142857 0.18571429 0.2 0.21428571 0.22857143 0.24285714 0.25714286 0.27142857 0.28571429 0.3 0.31428571 0.32857143 0.34285714 0.35714286 0.37142857 0.38571429 0.4 0.41428571 0.42857143 0.44285714 0.45714286 0.47142857 0.48571429 0.5 0.51428571 0.52857143 0.54285714 0.55714286 0.57142857 0.58571429 0.6 0.61428571 0.62857143 0.64285714 0.65714286 0.67142857 0.68571429 0.7 0.71428571 0.72857143 0.74285714 0.75714286 0.77142857 0.78571429 0.8 0.81428571 0.82857143 0.84285714 0.85714286 0.87142857 0.88571429 0.9 0.91428571 0.92857143 0.94285714 0.95714286 0.97142857 0.98571429 1 1 1 1 1 1
  line L27 (-18.5867, -15.5033) -> (-18.0673, -15.0704)
  arc A55 (-16.687, -15.166) -> (-18.0673, -15.0704) centre (-17.4271, -15.8386) ccw
  arc A56 (-16.687, -15.166) -> (-16.1839, -15.7018) centre (0, 0) ccw
  arc A57 (-16.1752, -17.0854) -> (-16.1839, -15.7018) centre (-16.9016, -16.3982) ccw
  line L28 (-16.1752, -17.0854) -> (-16.6398, -17.5766)
  spline S28 degree 5 poles (-16.6398, -17.5766) (-16.6454, -17.5825) (-16.6564, -17.5944) (-16.6726, -17.6127) (-16.6934, -17.6377) (-16.7184, -17.6698) (-16.7427, -17.7026) (-16.7664, -17.7358) (-16.79, -17.7693) (-16.8133, -17.8029) (-16.8365, -17.8366) (-16.8594, -17.8706) (-16.8821, -17.9048) (-16.9044, -17.9393) (-16.9263, -17.9741) (-16.9479, -18.0092) (-16.9691, -18.0445) (-16.9902, -18.0801) (-17.011, -18.1158) (-17.0316, -18.1517) (-17.052, -18.1878) (-17.0722, -18.224) (-17.0922, -18.2604) (-17.1119, -18.297) (-17.1314, -18.3338) (-17.1507, -18.3707) (-17.1698, -18.4078) (-17.1886, -18.4451) (-17.2073, -18.4825) (-17.2258, -18.5201) (-17.2441, -18.5578) (-17.2622, -18.5956) (-17.2802, -18.6336) (-17.2979, -18.6717) (-17.3155, -18.71) (-17.3328, -18.7484) (-17.35, -18.7869) (-17.367, -18.8256) (-17.3838, -18.8644) (-17.4005, -18.9033) (-17.417, -18.9424) (-17.4333, -18.9815) (-17.4494, -19.0208) (-17.4654, -19.0602) (-17.4812, -19.0998) (-17.4968, -19.1394) (-17.5123, -19.1792) (-17.5276, -19.219) (-17.5428, -19.259) (-17.5578, -19.2991) (-17.5726, -19.3393) (-17.5873, -19.3796) (-17.6018, -19.42) (-17.6161, -19.4606) (-17.6303, -19.5012) (-17.6444, -19.5419) (-17.6582, -19.5828) (-17.672, -19.6237) (-17.6855, -19.6647) (-17.699, -19.7058) (-17.7122, -19.7471) (-17.7254, -19.7884) (-17.7383, -19.8298) (-17.7512, -19.8713) (-17.7638, -19.9129) (-17.7764, -19.9546) (-17.7887, -19.9964) (-17.801, -20.0383) (-17.8131, -20.0803) (-17.825, -20.1223) (-17.8368, -20.1645) (-17.8461, -20.1982) (-17.853, -20.2236) (-17.8576, -20.2406) (-17.8599, -20.249) knots 0 0 0 0 0 0 0.01428571 0.02857143 0.04285714 0.05714286 0.07142857 0.08571429 0.1 0.11428571 0.12857143 0.14285714 0.15714286 0.17142857 0.18571429 0.2 0.21428571 0.22857143 0.24285714 0.25714286 0.27142857 0.28571429 0.3 0.31428571 0.32857143 0.34285714 0.35714286 0.37142857 0.38571429 0.4 0.41428571 0.42857143 0.44285714 0.45714286 0.47142857 0.48571429 0.5 0.51428571 0.52857143 0.54285714 0.55714286 0.57142857 0.58571429 0.6 0.61428571 0.62857143 0.64285714 0.65714286 0.67142857 0.68571429 0.7 0.71428571 0.72857143 0.74285714 0.75714286 0.77142857 0.78571429 0.8 0.81428571 0.82857143 0.84285714 0.85714286 0.87142857 0.88571429 0.9 0.91428571 0.92857143 0.94285714 0.95714286 0.97142857 0.98571429 1 1 1 1 1 1
  arc A58 (-17.8599, -20.249) -> (-16.5438, -21.3379) centre (0, 0) ccw
  spline S29 degree 5 poles (-14.1473, -19.6386) (-14.152, -19.6452) (-14.1617, -19.6583) (-14.1766, -19.6776) (-14.1972, -19.7027) (-14.2241, -19.7333) (-14.2518, -19.7632) (-14.28, -19.7928) (-14.3084, -19.8222) (-14.337, -19.8514) (-14.3658, -19.8805) (-14.3949, -19.9094) (-14.4242, -19.9381) (-14.454, -19.9664) (-14.4841, -19.9945) (-14.5145, -20.0222) (-14.5452, -20.0498) (-14.5762, -20.0771) (-14.6074, -20.1042) (-14.6388, -20.1312) (-14.6704, -20.158) (-14.7022, -20.1846) (-14.7342, -20.2111) (-14.7665, -20.2373) (-14.7989, -20.2634) (-14.8316, -20.2892) (-14.8645, -20.3149) (-14.8975, -20.3405) (-14.9308, -20.3658) (-14.9642, -20.391) (-14.9978, -20.4161) (-15.0316, -20.4409) (-15.0656, -20.4657) (-15.0997, -20.4902) (-15.134, -20.5146) (-15.1685, -20.5389) (-15.2031, -20.563) (-15.2379, -20.587) (-15.2729, -20.6108) (-15.308, -20.6344) (-15.3432, -20.6579) (-15.3787, -20.6813) (-15.4142, -20.7045) (-15.4499, -20.7276) (-15.4858, -20.7505) (-15.5218, -20.7733) (-15.558, -20.7959) (-15.5943, -20.8185) (-15.6307, -20.8408) (-15.6673, -20.8631) (-15.704, -20.8852) (-15.7408, -20.9071) (-15.7778, -20.9289) (-15.8149, -20.9506) (-15.8522, -20.9722) (-15.8896, -20.9936) (-15.9271, -21.0149) (-15.9647, -21.0361) (-16.0025, -21.0571) (-16.0403, -21.078) (-16.0783, -21.0987) (-16.1165, -21.1194) (-16.1547, -21.1399) (-16.1931, -21.1603) (-16.2316, -21.1805) (-16.2702, -21.2006) (-16.3089, -21.2206) (-16.3478, -21.2405) (-16.3867, -21.2602) (-16.4258, -21.2798) (-16.465, -21.2993) (-16.4964, -21.3148) (-16.5201, -21.3263) (-16.5359, -21.334) (-16.5438, -21.3379) knots 0 0 0 0 0 0 0.01428571 0.02857143 0.04285714 0.05714286 0.07142857 0.08571429 0.1 0.11428571 0.12857143 0.14285714 0.15714286 0.17142857 0.18571429 0.2 0.21428571 0.22857143 0.24285714 0.25714286 0.27142857 0.28571429 0.3 0.31428571 0.32857143 0.34285714 0.35714286 0.37142857 0.38571429 0.4 0.41428571 0.42857143 0.44285714 0.45714286 0.47142857 0.48571429 0.5 0.51428571 0.52857143 0.54285714 0.55714286 0.57142857 0.58571429 0.6 0.61428571 0.62857143 0.64285714 0.65714286 0.67142857 0.68571429 0.7 0.71428571 0.72857143 0.74285714 0.75714286 0.77142857 0.78571429 0.8 0.81428571 0.82857143 0.84285714 0.85714286 0.87142857 0.88571429 0.9 0.91428571 0.92857143 0.94285714 0.95714286 0.97142857 0.98571429 1 1 1 1 1 1
  line L29 (-14.1473, -19.6386) -> (-13.7518, -19.0901)
  arc A59 (-12.3912, -18.8395) -> (-13.7518, -19.0901) centre (-12.9407, -19.675) ccw
  arc A60 (-12.3912, -18.8395) -> (-11.7706, -19.2333) centre (0, 0) ccw
  arc A61 (-11.418, -20.5712) -> (-11.7706, -19.2333) centre (-12.2926, -20.0863) ccw
  line L30 (-11.418, -20.5712) -> (-11.7459, -21.1625)
  spline S30 degree 5 poles (-11.7459, -21.1625) (-11.7499, -21.1696) (-11.7576, -21.1839) (-11.7687, -21.2057) (-11.7827, -21.235) (-11.7989, -21.2724) (-11.8142, -21.3102) (-11.829, -21.3483) (-11.8434, -21.3865) (-11.8577, -21.4248) (-11.8717, -21.4633) (-11.8855, -21.5019) (-11.899, -21.5407) (-11.912, -21.5796) (-11.9245, -21.6188) (-11.9367, -21.6582) (-11.9485, -21.6977) (-11.96, -21.7374) (-11.9713, -21.7771) (-11.9823, -21.817) (-11.9931, -21.857) (-12.0037, -21.8971) (-12.014, -21.9374) (-12.024, -21.9777) (-12.0338, -22.0182) (-12.0433, -22.0588) (-12.0525, -22.0995) (-12.0615, -22.1402) (-12.0703, -22.1811) (-12.0789, -22.2221) (-12.0872, -22.2632) (-12.0954, -22.3043) (-12.1033, -22.3456) (-12.111, -22.3869) (-12.1185, -22.4284) (-12.1257, -22.4699) (-12.1328, -22.5115) (-12.1396, -22.5532) (-12.1463, -22.5949) (-12.1528, -22.6368) (-12.159, -22.6787) (-12.1651, -22.7207) (-12.1709, -22.7628) (-12.1766, -22.8049) (-12.1821, -22.8471) (-12.1874, -22.8894) (-12.1925, -22.9318) (-12.1974, -22.9742) (-12.2021, -23.0167) (-12.2067, -23.0592) (-12.211, -23.1019) (-12.2152, -23.1446) (-12.2192, -23.1873) (-12.223, -23.2301) (-12.2267, -23.273) (-12.2301, -23.3159) (-12.2334, -23.3589) (-12.2366, -23.402) (-12.2395, -23.4451) (-12.2423, -23.4883) (-12.2449, -23.5315) (-12.2473, -23.5748) (-12.2496, -23.6182) (-12.2517, -23.6616) (-12.2536, -23.705) (-12.2554, -23.7485) (-12.257, -23.7921) (-12.2584, -23.8357) (-12.2597, -23.8793) (-12.2608, -23.923) (-12.2617, -23.9668) (-12.2624, -24.0018) (-12.2627, -24.0281) (-12.263, -24.0457) (-12.2631, -24.0545) knots 0 0 0 0 0 0 0.01428571 0.02857143 0.04285714 0.05714286 0.07142857 0.08571429 0.1 0.11428571 0.12857143 0.14285714 0.15714286 0.17142857 0.18571429 0.2 0.21428571 0.22857143 0.24285714 0.25714286 0.27142857 0.28571429 0.3 0.31428571 0.32857143 0.34285714 0.35714286 0.37142857 0.38571429 0.4 0.41428571 0.42857143 0.44285714 0.45714286 0.47142857 0.48571429 0.5 0.51428571 0.52857143 0.54285714 0.55714286 0.57142857 0.58571429 0.6 0.61428571 0.62857143 0.64285714 0.65714286 0.67142857 0.68571429 0.7 0.71428571 0.72857143 0.74285714 0.75714286 0.77142857 0.78571429 0.8 0.81428571 0.82857143 0.84285714 0.85714286 0.87142857 0.88571429 0.9 0.91428571 0.92857143 0.94285714 0.95714286 0.97142857 0.98571429 1 1 1 1 1 1
  arc A62 (-12.2631, -24.0545) -> (-10.7175, -24.7818) centre (0, 0) ccw
  spline S31 degree 5 poles (-8.8189, -22.5399) (-8.8218, -22.5475) (-8.8279, -22.5625) (-8.8376, -22.585) (-8.8513, -22.6144) (-8.8698, -22.6507) (-8.8891, -22.6866) (-8.909, -22.7223) (-8.9293, -22.7578) (-8.9498, -22.7932) (-8.9704, -22.8286) (-8.9914, -22.8638) (-9.0127, -22.8988) (-9.0344, -22.9337) (-9.0566, -22.9684) (-9.0792, -23.0028) (-9.1021, -23.0371) (-9.1253, -23.0713) (-9.1488, -23.1053) (-9.1725, -23.1393) (-9.1964, -23.1731) (-9.2206, -23.2068) (-9.245, -23.2403) (-9.2697, -23.2738) (-9.2947, -23.3071) (-9.3199, -23.3403) (-9.3454, -23.3733) (-9.371, -23.4063) (-9.3969, -23.4391) (-9.4231, -23.4718) (-9.4494, -23.5045) (-9.4759, -23.537) (-9.5026, -23.5694) (-9.5296, -23.6016) (-9.5567, -23.6338) (-9.5841, -23.6659) (-9.6117, -23.6978) (-9.6394, -23.7297) (-9.6673, -23.7614) (-9.6955, -23.7931) (-9.7238, -23.8246) (-9.7523, -23.8561) (-9.781, -23.8874) (-9.8098, -23.9186) (-9.8389, -23.9498) (-9.8681, -23.9808) (-9.8974, -24.0117) (-9.927, -24.0425) (-9.9567, -24.0733) (-9.9866, -24.1039) (-10.0167, -24.1344) (-10.0469, -24.1649) (-10.0773, -24.1952) (-10.1079, -24.2254) (-10.1386, -24.2556) (-10.1695, -24.2856) (-10.2005, -24.3156) (-10.2317, -24.3454) (-10.263, -24.3752) (-10.2945, -24.4048) (-10.3262, -24.4344) (-10.358, -24.4639) (-10.3899, -24.4932) (-10.422, -24.5225) (-10.4543, -24.5517) (-10.4867, -24.5808) (-10.5192, -24.6098) (-10.5519, -24.6387) (-10.5847, -24.6675) (-10.6177, -24.6962) (-10.6508, -24.7248) (-10.6774, -24.7476) (-10.6974, -24.7647) (-10.7108, -24.7761) (-10.7175, -24.7818) knots 0 0 0 0 0 0 0.01428571 0.02857143 0.04285714 0.05714286 0.07142857 0.08571429 0.1 0.11428571 0.12857143 0.14285714 0.15714286 0.17142857 0.18571429 0.2 0.21428571 0.22857143 0.24285714 0.25714286 0.27142857 0.28571429 0.3 0.31428571 0.32857143 0.34285714 0.35714286 0.37142857 0.38571429 0.4 0.41428571 0.42857143 0.44285714 0.45714286 0.47142857 0.48571429 0.5 0.51428571 0.52857143 0.54285714 0.55714286 0.57142857 0.58571429 0.6 0.61428571 0.62857143 0.64285714 0.65714286 0.67142857 0.68571429 0.7 0.71428571 0.72857143 0.74285714 0.75714286 0.77142857 0.78571429 0.8 0.81428571 0.82857143 0.84285714 0.85714286 0.87142857 0.88571429 0.9 0.91428571 0.92857143 0.94285714 0.95714286 0.97142857 0.98571429 1 1 1 1 1 1
  line L31 (-8.8189, -22.5399) -> (-8.5723, -21.9103)
  arc A63 (-7.3167, -21.3292) -> (-8.5723, -21.9103) centre (-7.6412, -22.275) ccw
  arc A64 (-7.3167, -21.3292) -> (-6.6176, -21.5563) centre (0, 0) ccw
  arc A65 (-5.9435, -22.7645) -> (-6.6176, -21.5563) centre (-6.9111, -22.5122) ccw
  line L32 (-5.9435, -22.7645) -> (-6.114, -23.4187)